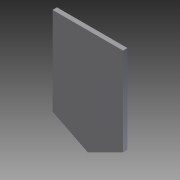
# Autodesk Inventor part: mean machine tooth
Saved by Autodesk Inventor 2012 (Build 160160000, 160)
## iProperties
Created: 2013-12-19
Part Number: mean machine tooth
Material: Default
Document SubType Name: Modeling
Designer: Bryce
Density: 1 g/cm^3
Author: Bryce
Autodesk Inventor part; units mm, degrees
ref_plane "YZ Plane" through (0, 0, 0) normal (1, 0, 0) x (0, 1, 0)
ref_plane "XZ Plane" through (0, 0, 0) normal (0, 1, 0) x (-1, 0, 0)
ref_plane "XY Plane" through (0, 0, 0) normal (0, 0, 1) x (1, 0, 0)
sketch "Sketch1" plane through (0, 0, 0) normal (0, 0, 1) x (1, 0, 0)
  line L0 (0, 0) -> (50.8, 0)
  line L1 (50.8, 0) -> (50.8, -63.5)
  line L2 (50.8, -63.5) -> (25.4, -76.2)
  line L3 (25.4, -76.2) -> (0, -63.5)
  line L4 (0, -63.5) -> (0, 0)
  dimension "d0" = 50.8
  dimension "d1" = 76.2
  dimension "d2" = 63.5
  constraints: 10 end point, 2 equal length, 1 horizontal, 1 parallel, 1 perpendicular
  measures "d0" distance of L0.start L0.end
  measures "d1" distance from line of L2.end L0
  measures "d2" distance of L3.end L0.start
extrude "Extrusion1" add sketch "Sketch1" along normal blind 3.175
body "Solid1"
